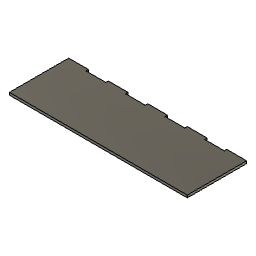
side (Autodesk Fusion 360 design; units mm, degrees)
Autodesk Fusion 360 part; units mm, degrees
sketch "Sketch1" plane through (0, 0, 0) normal (0, 0, 1) x (1, 0, 0)
  line L0 (-114.3, 0) -> (114.3, 0)
  line L1 (114.3, 0) -> (114.3, -76.2)
  line L2 (114.3, -76.2) -> (-114.3, -76.2)
  line L3 (-114.3, -76.2) -> (-114.3, 0)
  dimension "d1" = 228.6
  dimension "d2" = 76.2
  dimension "d3" = 114.3
  constraint horizontal L0
  constraint vertical L1
  constraint horizontal L2
  constraint vertical L3
  constraint horizontal origin L0.start
  measures "d1" distance of L0.start L0.end
  measures "d2" distance of L0.start L2.end
  measures "d3" horizontal distance of origin L0.start
extrude "Extrude1" add sketch "Sketch1" along normal blind 3.175
sketch "Sketch2" plane through (0, 0, 3.175) normal (0, 0, 1) x (-1, 0, 0)
  line L0 (114.3, 76.2) -> (-114.3, 76.2)
  line L1 (-114.3, 76.2) -> (-114.3, 0)
  line L2 (-114.3, 0) -> (114.3, 0)
  line L3 (114.3, 0) -> (114.3, 76.2)
  line L4 (88.9, 0) -> (63.5, 0)
  line L5 (63.5, 0) -> (63.5, 3.175)
  line L6 (63.5, 3.175) -> (88.9, 3.175)
  line L7 (88.9, 3.175) -> (88.9, 0)
  dimension "d6" = 3.175
  dimension "d7" = 25.4
  dimension "d8" = 25.4
  constraint horizontal L4
  constraint vertical L5
  constraint horizontal L6
  constraint vertical L7
  constraint coincident L2 L4.start
  measures "d6" distance of L4.start L6.end
  measures "d7" distance of L4.start L4.end
  measures "d8" distance of L2.end L4.start
extrude "Extrude2" cut sketch "Sketch2" against normal through all contours L2 L4 L5 L6 L7
pattern_path "PathPattern1" count 4 spacing 50.8 from (-63.5, 0, 3.175) along 1 edges at (25.4, 0, 3.175) of "Extrude2"
